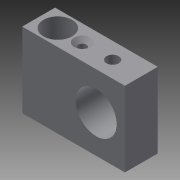
# Autodesk Inventor part: HeaterBlock
Saved by Autodesk Inventor 2014 SP1 (Build 180222100, 222)
## iProperties
Created: 2013-12-27
Part Number: HeaterBlock
Material: Generic
Document SubType Name: Modeling
Designer: Jack
Density: 1 g/cm^3
Appearance: Default
Author: Jack
Autodesk Inventor part; units mm, degrees
ref_plane "YZ Plane" through (0, 0, 0) normal (1, 0, 0) x (0, 1, 0)
ref_plane "XZ Plane" through (0, 0, 0) normal (0, 1, 0) x (-1, 0, 0)
ref_plane "XY Plane" through (0, 0, 0) normal (0, 0, 1) x (1, 0, 0)
sketch "Sketch1" plane through (0, 0, 0) normal (0, 1, 0) x (-1, 0, 0)
  line L0 (0, 0) -> (25, 0)
  line L1 (25, 0) -> (25, 18.26)
  line L2 (25, 18.26) -> (0, 18.26)
  line L3 (0, 18.26) -> (0, 0)
  dimension "d0" = 25
  dimension "d1" = 18.26
  constraints: 8 end point, 3 perpendicular, 1 horizontal
  measures "d0" distance of L0.start L0.end
  measures "d1" distance of L0.end L1.end
extrude "Extrusion1" add sketch "Sketch1" along normal blind 8
sketch "Sketch2" plane through (0, 8, 0) normal (0, 1, 0) x (1, 0, 0)
  line L0 (0, 0) -> (-25, 0) projected
  line L1 (0, -18.26) -> (0, 0) projected
  circle A0 centre (-7, -9.13) radius 5
  dimension "d4" = 10
  dimension "d5" = 7
  dimension "d6" = 9.13
  constraints: 1 centre point
  measures "d4" diameter of A0
  measures "d5" distance from line of L1 A0.centre
  measures "d6" distance from line of L0 A0.centre
extrude "Extrusion2" cut sketch "Sketch2" against normal blind 8
sketch "Sketch3" plane through (-25, 0, 18.26) normal (0, 0, 1) x (1, 0, 0)
  line L0 (0, 0) -> (25, 0) projected
  line L1 (25, 0) -> (25, 8) projected
  circle A0 centre (4.66, 4) radius 3.5
  circle A1 centre (10.64, 4) radius 0.9905
  dimension "d9" = 7
  dimension "d10" = 1.981
  dimension "d13" = 14.36
  dimension "d14" = 20.34
  dimension "d15" = 4
  constraints: 2 centre point, 1 horizontal alignment
  measures "d9" diameter of A0
  measures "d10" diameter of A1
  measures "d13" distance from line of L1 A1.centre
  measures "d14" distance from line of L1 A0.centre
  measures "d15" distance from line of L0 A0.centre
extrude "Extrusion3" cut sketch "Sketch3" against normal blind 18.5
sketch "Sketch4" plane through (-25, 0, 18.26) normal (0, 0, 1) x (1, 0, 0)
  line L0 (0, 0) -> (25, 0) projected
  line L1 (25, 0) -> (25, 8) projected
  circle A0 centre (18, 4) radius 1.5
  dimension "d18" = 3
  dimension "d19" = 7
  dimension "d20" = 4
  constraints: 1 centre point
  measures "d18" diameter of A0
  measures "d19" distance from line of L1 A0.centre
  measures "d20" distance from line of L0 A0.centre
extrude "Extrusion4" cut sketch "Sketch4" against normal blind 6.5
chamfer "Chamfer1" distance 1 angle 45 2 edges at (-15.3505, 4, 18.26) (-15.3505, 4, 0)
body "Solid1"
